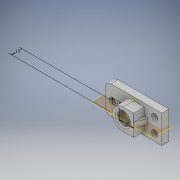
# Autodesk Inventor part: Деталь_5
Saved by Autodesk Inventor 2019.3 (Build 233278000, 278)
## iProperties
Created: 2020-03-23
Part Number: Деталь_5
Material: Типовые
Document SubType Name: Modeling
Designer: Diana
Density: 1 g/cm^3
Appearance: По умолчанию
Author: Diana
Autodesk Inventor part; units mm, degrees
ref_plane "YZ Plane" through (0, 0, 0) normal (1, 0, 0) x (0, 1, 0)
ref_plane "XY Plane" through (0, 0, 0) normal (0, 0, 1) x (1, 0, 0)
sketch "Эскиз1" plane through (0, 0, 0) normal (0, 0, 1) x (1, 0, 0)
  line L0 (40, -20) -> (-32, -20)
  line L1 (-40, -12) -> (-40, 12)
  line L2 (-32, 20) -> (40, 20)
  line L3 (40, 20) -> (40, -20)
  line L4 (40, -20) -> (-40, 20) construction
  line L5 (-40, -20) -> (40, 20) construction
  line L6 (-57.9882, 0) -> (56.3314, 0) projected
  arc A0 (-32, 20) -> (-40, 12) centre (-32, 12) ccw
  arc A1 (-40, -12) -> (-32, -20) centre (-32, -12) ccw
  point P0 (0, 0)
  dimension "d0" = 80
  dimension "d1" = 40
  dimension "d2" = 8
  dimension "d3" = 8
  constraints: 12 end point, 4 point on circle, 4 point on line, 4 tangent, 2 centre point, 2 midpoint, 2 parallel, 1 horizontal, 1 perpendicular, 1 other
  measures "d0" distance of L0.start L5.start
  measures "d1" distance of L0.start L2.end
  measures "d2" radius of A0
  measures "d3" radius of A1
extrude "Выдавливание1" add sketch "Эскиз1" along normal blind 10
sketch "Эскиз2" plane through (0, 0, 10) normal (0, 0, 1) x (1, 0, 0)
  line L0 (-57.9882, 0) -> (56.3314, 0) projected
  line L1 (-32, -20) -> (40, -20) projected
  line L2 (40, -20) -> (40, 20) projected
  line L3 (40, 20) -> (-32, 20) projected
  arc A0 (-32, 20) -> (-40, 12) centre (-32, 12) ccw projected
  line L4 (-40, 12) -> (-40, -12) projected
  arc A1 (-40, -12) -> (-32, -20) centre (-32, -12) ccw projected
  line L5 (0, -15) -> (15, -15)
  line L6 (15, -15) -> (15, 15)
  line L7 (15, 15) -> (0, 15)
  line L8 (0, 15) -> (0, -15)
  arc A2 (0, 15) -> (0, -15) centre (0, 0) ccw
  point P0 (0, 0)
  dimension "d6" = 30
  dimension "d7" = 15
  dimension "d8" = 15
  constraints: 8 end point, 2 midpoint, 2 parallel, 2 point on circle, 1 centre point, 1 horizontal, 1 perpendicular
  measures "d6" distance of L5.end L6.end
  measures "d7" distance of L5.start L5.end
  measures "d8" radius of A2
extrude "Выдавливание2" add sketch "Эскиз2" along normal blind 15 contours A2 L8 L0 | L0 L8 A2 | L8 L7 L6 L0 | L0 L6 L5 L8
sketch "Эскиз3" plane through (0, 0, 25) normal (0, 0, 1) x (1, 0, 0)
  arc A0 (0, 15) -> (0, -15) centre (0, 0) ccw projected
  line L0 (0, -15) -> (15, -15) projected
  line L1 (15, -15) -> (15, 15) projected
  line L2 (15, 15) -> (0, 15) projected
  point P0 (0, 0)
hole "Отверстие1" at (0, 0, 25) direction (0, 0, -1) diameter 18.376 depth 20 thread size "M20x1.5" class "6H" standard "ISO Metric profile"
chamfer "Фаска1" distance 1.6 angle 45 1 edges at (0, 9.188, 25)
sketch "Эскиз4" plane through (0, 0, 10) normal (0, 0, 1) x (1, 0, 0)
  line L0 (-56, 0) -> (56, 0) projected
  point P0 (0, 0)
  point P1 (-30, 0)
  point P2 (30, 10)
  point P3 (30, -10)
  dimension "d21" = 30
  dimension "d22" = 30
  dimension "d23" = 20
  constraints: 1 point on line, 1 symmetric about line
  measures "d21" distance of point (0, 0) point (-30, 0)
  measures "d22" horizontal distance of point (30, -10) point (0, 0)
  measures "d23" distance of point (30, -10) point (30, 10)
hole "Отверстие2" at (-30, 0, 10) at (30, 10, 10) at (30, -10, 10) direction (0, 0, -1) diameter 9 end through all
sketch "Эскиз5" plane through (0, 0, 0) normal (0, 1, 0) x (-1, 0, 0)
  line L0 (-15, 25) -> (-20, 10)
  point P0 (0, 0)
  point P1 (-15, 10)
  dimension "d31" = 5
  constraints: 2 end point, 1 coincident, 1 horizontal alignment
  measures "d31" distance of L0.end point (-15, 10)
extrude "Ребро жесткости1" add sketch "Эскиз5" along normal mid plane 7 rib yes fills toward (-17.4526, 17.4842) open curves L0
sketch "Эскиз6" plane through (0, 0, 10) normal (0, 0, 1) x (1, 0, 0)
  point P0 (0, 0)
sketch "Эскиз7" plane through (0, 0, 10) normal (0, 0, 1) x (1, 0, 0)
  arc A0 (0, 15) -> (0, -15) centre (0, 0) ccw projected
  line L0 (-20, 3.5) -> (-14.586, 3.5)
  line L1 (-14.586, 3.5) -> (-14.586, -3.5)
  line L2 (-14.586, -3.5) -> (-20, -3.5)
  line L3 (-20, -3.5) -> (-20, 3.5)
  point P0 (0, 0)
  dimension "d38" = 7
  dimension "d39" = 20
  constraints: 8 end point, 2 parallel, 2 point on circle, 1 horizontal, 1 perpendicular
  measures "d38" distance of L2.end L0.start
  measures "d39" distance from line of L3 point (0, 0)
sketch "Эскиз8" plane through (0, 0, 0) normal (0, 1, 0) x (-1, 0, 0)
  line L0 (20, 10) -> (15, 25)
  point P0 (0, 0)
  dimension "d41" = 15
  constraints: 2 end point, 1 coincident
  measures "d41" vertical distance of L0.end point (20, 10)
